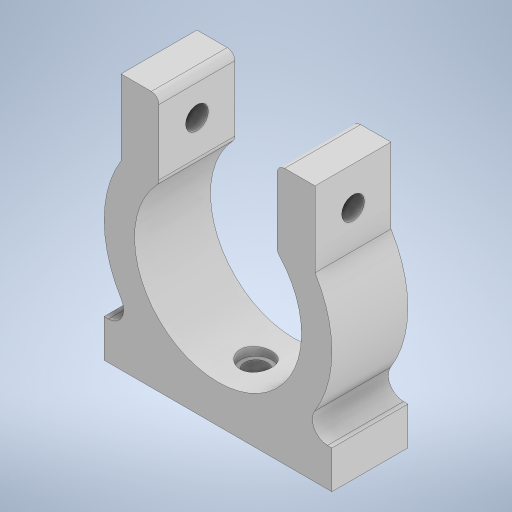
# Autodesk Inventor part: buisClip
Saved by Autodesk Inventor 2023 (Build 270158000, 158)
## iProperties
Created: 2023-09-25
Part Number: buisClip
Material: Generic
Document SubType Name: Modeling
Designer: Nikita
Density: 1 g/cm^3
Appearance: Default
Author: Nikita
Autodesk Inventor part; units mm, degrees
ref_plane "YZ Plane" through (0, 0, 0) normal (1, 0, 0) x (0, 1, 0)
ref_plane "XZ Plane" through (0, 0, 0) normal (0, 1, 0) x (-1, 0, 0)
ref_plane "XY Plane" through (0, 0, 0) normal (0, 0, 1) x (1, 0, 0)
sketch "Sketch1" plane through (0, 0, 0) normal (0, 0, 1) x (1, 0, 0)
  arc A0 (-7.7782, 7.7782) -> (7.7782, 7.7782) centre (0, 0) ccw
  line L0 (7.7782, 7.7782) -> (11.0228, 11.0228)
  line L1 (0, 0) -> (15.5887, 0) construction
  line L2 (0, 0) -> (20, 0) construction
  line L3 (-7.7782, 7.7782) -> (-10.6066, 10.6066)
  line L4 (15, -11) -> (15, -16)
  line L5 (15, -16) -> (-15, -16)
  line L6 (-15, -16) -> (-15, -11)
  line L7 (-15, -11) -> (-10.198, -11)
  arc A1 (-10.6066, 10.6066) -> (-10.198, -11) centre (0, 0) ccw
  arc A2 (10.198, -11) -> (10.6066, 10.6066) centre (0, 0) ccw
  line L8 (15, -11) -> (10.198, -11)
  dimension "d6" = 5
  dimension "d7" = 30
  constraints: 18 end point, 6 point on circle, 3 centre point, 3 horizontal, 3 perpendicular, 2 coincident, 1 point on line, 1 tangent
  measures "d6" distance of L4.start L4.end
  measures "d7" distance of L4.end L5.end
extrude "Extrusion1" add sketch "Sketch1" along normal blind 10
sketch "Sketch2" plane through (-15, -16, 0) normal (0, -1, 0) x (1, 0, 0)
  line L0 (0, 10) -> (30, 10) projected
  line L1 (30, 10) -> (25.198, 10) projected
  line L2 (0, 0) -> (30, 0) projected
  circle A0 centre (15, 5) radius 1.5
  point P0 (15, 0)
  dimension "d10" = 3
  constraints: 1 centre point
  measures "d10" diameter of A0
extrude "Extrusion2" cut sketch "Sketch2" against normal blind 24.75
sketch "Sketch3" plane through (10.198, -11, 0) normal (0, 1, 0) x (1, 0, 0)
  line L0 (4.802, 0) -> (0, 0) projected
  line L1 (-20.3961, -10) -> (-25.198, -10) projected
  line L2 (-20.3961, 0) -> (-25.198, 0) projected
  line L3 (4.802, -10) -> (0, -10) projected
  circle A0 centre (-10.198, -5) radius 2.0833
  point P0 (-10.198, 0)
  constraints: 1 centre point
sketch "Sketch4" plane through (0, 0, 0) normal (0, 0, -1) x (-1, 0, 0)
  point P0 (0, 0)
extrude "Extrusion3" cut sketch "Sketch3" against normal blind 1
sketch "Sketch5" plane through (10.198, -11, 0) normal (0, -1, 0) x (1, 0, 0)
  arc A0 (-10.198, 3.5) -> (-10.198, 6.5) centre (-10.198, 5) ccw projected
  arc A1 (-10.198, 2.9167) -> (-10.198, 7.0833) centre (-10.198, 5) ccw projected
  circle A2 centre (-10.198, 5) radius 2.0833
  point P0 (-10.198, 0)
  point P1 (-10.198, 2.9167)
  constraints: 1 coincident, 3 other
extrude "Extrusion4" cut sketch "Sketch5" against normal blind 1.5
fillet "Fillet1" radius 2 1 edges at (-10.198, -11, 5)
fillet "Fillet2" radius 2 1 edges at (10.198, -11, 5)
sketch "Sketch6" plane through (0, 0, 10) normal (0, 0, 1) x (1, 0, 0)
  line L0 (-7.7782, 7.7782) -> (-10.6066, 10.6066) projected
  line L1 (-7.7782, 7.7782) -> (-7.7782, 17.7782)
  line L2 (-7.7782, 17.7782) -> (-12.7782, 17.7782)
  line L3 (-12.7782, 17.7782) -> (-12.7782, 7.8561)
  arc A0 (-10.6066, 10.6066) -> (-12.7255, -7.9412) centre (0, 0) ccw projected
  dimension "d21" = 10
  dimension "d22" = 5
  constraints: 6 end point, 1 horizontal, 1 perpendicular, 1 point on circle, 1 vertical
  measures "d21" distance of L0.start L1.end
  measures "d22" distance of L1.end L2.end
extrude "Extrusion5" add sketch "Sketch6" against normal blind 10
sketch "Sketch7" plane through (0, 0, 10) normal (0, 0, 1) x (1, 0, 0)
  line L0 (7.7782, 7.7782) -> (7.7782, 17.7782)
  line L1 (7.7782, 17.7782) -> (12.7782, 17.7782)
  line L2 (12.7782, 17.7782) -> (12.7782, 7.8561)
  arc A0 (12.7255, -7.9412) -> (10.6066, 10.6066) centre (0, 0) ccw projected
  arc A1 (-7.7782, 7.7782) -> (7.7782, 7.7782) centre (0, 0) ccw projected
  line L3 (7.7782, 7.7782) -> (12.7782, 7.8561)
  dimension "d25" = 5
  constraints: 8 end point, 2 perpendicular, 1 point on circle, 1 vertical
  measures "d25" distance of L0.end L1.end
extrude "Extrusion6" add sketch "Sketch7" against normal blind 10
sketch "Sketch8" plane through (12.7782, 7.8561, 10) normal (1, 0, 0) x (0, 0, -1)
  line L0 (0, 9.9221) -> (0, 0) construction
  line L1 (10, -0.0779) -> (0, -0.0779) construction
  line L2 (0, 9.9221) -> (10, -0.0779) construction
  line L3 (0, 9.9221) -> (10, 9.9221) construction
  line L4 (10, 9.9221) -> (0, -0.0779) construction
  circle A0 centre (5, 4.9221) radius 1.5
  point P0 (10, -7.8561)
  dimension "d28" = 3
  constraints: 4 end point, 1 centre point, 1 midpoint
  measures "d28" diameter of A0
extrude "Extrusion7" cut sketch "Sketch8" against normal blind 36
fillet "Fillet5" radius 1 1 edges at (-7.7782, 17.7782, 5)
fillet "Fillet6" radius 1 1 edges at (-7.7782, 7.7782, 5)
fillet "Fillet7" radius 1 1 edges at (7.7782, 17.7782, 5)
fillet "Fillet8" radius 1 1 edges at (7.7782, 7.7782, 5)
body "Solid1"
